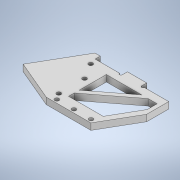
# Autodesk Inventor part: Trunk_lower_side_frame
Saved by Autodesk Inventor 2020.4 (Build 244396000, 396)
## iProperties
Created: 2022-01-02
Part Number: Trunk_lower_side_frame
Material: 一般
Document SubType Name: Modeling
Designer: Masato Kubotera
Density: 1 g/cm^3
Appearance: 既定
Mass: 14.6824 g
Surface Area: 92.1199 cm^2
Volume: 14.6824 cm^3
Author: Masato Kubotera
Autodesk Inventor part; units mm, degrees
ref_plane "YZ Plane" through (0, 0, 0) normal (1, 0, 0) x (0, 1, 0)
ref_plane "XZ Plane" through (0, 0, 0) normal (0, 1, 0) x (-1, 0, 0)
ref_plane "XY Plane" through (0, 0, 0) normal (0, 0, 1) x (1, 0, 0)
derived "Trunk_basis.ipt"
sketch "スケッチ1" plane through (0, 0, 0) normal (0, 1, 0) x (-1, 0, 0)
  line L0 (0, 22) -> (0, -143) construction
  circle A0 centre (5, 0) radius 10.5 construction
  line L1 (-7, 16) -> (36, 16) construction
  line L2 (36, 16) -> (36, -16) construction
  line L3 (36, -16) -> (-7, -16) construction
  line L4 (-7, -16) -> (-7, 16) construction
  line L5 (-7, 16) -> (36, -16) construction
  line L6 (36, 16) -> (-7, -16) construction
  line L7 (33, 13.5) -> (6, 13.5) construction
  line L8 (6, 13.5) -> (6, -13.5) construction
  line L9 (6, -13.5) -> (33, -13.5) construction
  line L10 (33, -13.5) -> (33, 13.5) construction
  line L11 (33, 13.5) -> (6, -13.5) construction
  line L12 (6, 13.5) -> (33, -13.5) construction
  line L13 (-7, 0) -> (36, 0) construction
  arc A1 (5, 16) -> (-7, 10.583) centre (5, 0) ccw construction
  line L14 (34.5651, -16.05) -> (5, -16.05)
  line L15 (5, 16.05) -> (34.5651, 16.05)
  line L16 (36.05, 14.5651) -> (36.05, -14.5651)
  line L17 (36.05, -16.05) -> (-7.05, 16.05) construction
  line L18 (-7.05, -16.05) -> (36.05, 16.05) construction
  arc A2 (5, 16.05) -> (-6.5314, 11.1638) centre (5, 0) ccw
  arc A3 (-6.5314, 11.1638) -> (-7.05, 9.8372) centre (-6.0721, 10.2196) ccw
  arc A4 (36.05, 14.5651) -> (34.5651, 16.05) centre (35.3075, 15.3075) ccw
  circle A5 centre (6, 13.5) radius 1.35 construction
  line L19 (19.5, 13.5) -> (19.5, -13.5) construction
  circle A6 centre (33, 13.5) radius 1.35 construction
  line L20 (-12, 22) -> (-14.5, 19.5)
  line L21 (-14.5, 19.5) -> (-14.5, -13.5)
  line L22 (-14.5, -13.5) -> (-28.5, -27.5)
  line L23 (-28.5, -27.5) -> (-28.5, -97)
  line L24 (52, -13.5) -> (52, 19.5)
  line L25 (52, 19.5) -> (49.5, 22)
  line L26 (49.5, 22) -> (-12, 22)
  line L27 (-28.5, -121.925) -> (-28.5, -139)
  line L28 (-16, -139) -> (-16, -99.5) construction
  line L29 (-16, -99.5) -> (16, -99.5) construction
  line L30 (16, -139) -> (16, -99.5) construction
  line L31 (-7.5, -139) -> (-7.5, -143)
  line L32 (-7.5, -143) -> (7.5, -143)
  line L33 (7.5, -139) -> (7.5, -143)
  arc A7 (-7.5, -139) -> (-9.6, -139) centre (-8.55, -139) ccw
  arc A8 (9.6, -139) -> (7.5, -139) centre (8.55, -139) ccw
  line L34 (-22, -139) -> (-22, -133) construction
  line L35 (-23.5, -133) -> (-20.5, -133) construction
  line L36 (-23.5, -133) -> (-23.5, -139) construction
  line L37 (-20.5, -133) -> (-20.5, -139) construction
  line L38 (-12, 22) -> (-7, 22) construction
  line L39 (-7, 22) -> (-7, -22) construction
  line L40 (-7, -22) -> (-12, -22) construction
  line L41 (-12, -22) -> (-12, 22) construction
  line L42 (-12, 22) -> (-7, -22) construction
  line L43 (-7, 22) -> (-12, -22) construction
  line L44 (-9.5, 22) -> (-9.5, -22) construction
  line L45 (-7, 0) -> (-12, 0) construction
  circle A9 centre (-9.5, 17.75) radius 1.6
  line L46 (-12, 10) -> (-9.5, 10) construction
  line L47 (-9.5, 10) -> (-9.5, -10) construction
  line L48 (-9.5, -10) -> (-12, -10) construction
  line L49 (-12, -10) -> (-12, 10) construction
  line L50 (-12, 10) -> (-9.5, -10) construction
  line L51 (-9.5, 10) -> (-12, -10) construction
  line L52 (-9.45, 10.05) -> (-12.05, 10.05)
  line L53 (-12.05, 7.95) -> (-12.05, -7.95)
  line L54 (-12.05, -10.05) -> (-9.45, -10.05)
  line L55 (-9.45, -7.95) -> (-9.45, 7.95)
  line L56 (-9.45, 10.05) -> (-12.05, -10.05) construction
  line L57 (-12.05, 10.05) -> (-9.45, -10.05) construction
  arc A10 (-12.05, 10.05) -> (-12.05, 7.95) centre (-12.05, 9) ccw
  line L58 (-10.75, 10) -> (-10.75, -10) construction
  arc A11 (-9.45, 7.95) -> (-9.45, 10.05) centre (-9.45, 9) ccw
  circle A12 centre (-9.5, -17.75) radius 1.6
  arc A13 (-12.05, -7.95) -> (-12.05, -10.05) centre (-12.05, -9) ccw
  arc A14 (-9.45, -10.05) -> (-9.45, -7.95) centre (-9.45, -9) ccw
  line L59 (36, 14.4) -> (44.5, 14.4) construction
  line L60 (44.5, 14.4) -> (44.5, -14.4) construction
  line L61 (36, -14.4) -> (44.5, -14.4) construction
  line L62 (46.95, 7.95) -> (46.95, -7.95)
  line L63 (49.5, 0) -> (44.5, 0) construction
  line L64 (44.5, 22) -> (49.5, 22) construction
  line L65 (49.55, -7.95) -> (49.55, 7.95)
  line L66 (48.25, 10) -> (48.25, -10) construction
  line L67 (49.5, 10) -> (47, -10) construction
  line L68 (49.5, -10) -> (47, -10) construction
  line L69 (49.5, 10) -> (49.5, -10) construction
  line L70 (47, 10) -> (49.5, -10) construction
  line L71 (46.95, -10.05) -> (49.55, -10.05)
  line L72 (46.95, 10.05) -> (49.55, -10.05) construction
  line L73 (49.55, 10.05) -> (46.95, -10.05) construction
  line L74 (49.5, -22) -> (44.5, -22) construction
  line L75 (44.5, 22) -> (49.5, -22) construction
  line L76 (49.5, 22) -> (49.5, -22) construction
  line L77 (49.5, 22) -> (44.5, -22) construction
  line L78 (47, 22) -> (47, -22) construction
  line L79 (44.5, -22) -> (44.5, 22) construction
  circle A15 centre (47, -17.75) radius 1.6
  arc A16 (49.55, -10.05) -> (49.55, -7.95) centre (49.55, -9) ccw
  line L80 (47, -10) -> (47, 10) construction
  arc A17 (46.95, -7.95) -> (46.95, -10.05) centre (46.95, -9) ccw
  arc A18 (46.95, 10.05) -> (46.95, 7.95) centre (46.95, 9) ccw
  arc A19 (49.55, 7.95) -> (49.55, 10.05) centre (49.55, 9) ccw
  line L81 (47, 10) -> (49.5, 10) construction
  line L82 (49.55, 10.05) -> (46.95, 10.05)
  circle A20 centre (47, 17.75) radius 1.6
  circle A21 centre (5, 0) radius 16 construction
  arc A22 (-6.5314, -11.1638) -> (5, -16.05) centre (5, 0) ccw
  arc A23 (-7.05, -9.8372) -> (-6.5314, -11.1638) centre (-6.0721, -10.2196) ccw
  arc A24 (34.5651, -16.05) -> (36.05, -14.5651) centre (35.3075, -15.3075) ccw
  line L83 (-7.05, -9.8372) -> (-7.05, 9.8372)
  line L84 (22, -139) -> (22, -133) construction
  line L85 (23.5, -133) -> (23.5, -139) construction
  line L86 (20.5, -133) -> (20.5, -139) construction
  line L87 (23.5, -133) -> (20.5, -133) construction
  circle A25 centre (6, -13.5) radius 1.35
  circle A26 centre (33, -13.5) radius 1.35
  line L88 (188, -110.7642) -> (183, -110.7642)
  line L89 (183, -110.7642) -> (183, -167.2358) construction
  line L90 (183, -167.2358) -> (188, -167.2358) construction
  line L91 (188, -167.2358) -> (188, -110.7642)
  line L92 (188, -110.7642) -> (183, -167.2358) construction
  line L93 (183, -110.7642) -> (188, -167.2358) construction
  line L94 (22, -108.5) -> (56, -108.5) construction
  line L95 (56, -108.5) -> (56, -131.5) construction
  line L96 (56, -131.5) -> (22, -131.5) construction
  line L97 (22, -131.5) -> (22, -108.5) construction
  line L98 (22, -108.5) -> (56, -131.5) construction
  line L99 (56, -108.5) -> (22, -131.5) construction
  line L100 (22, -131.5) -> (52, -131.5) construction
  line L101 (52, -131.5) -> (52, -136.5) construction
  line L102 (52, -136.5) -> (22, -136.5) construction
  line L103 (22, -136.5) -> (22, -131.5) construction
  line L104 (22, -131.5) -> (52, -136.5) construction
  line L105 (52, -131.5) -> (22, -136.5) construction
  line L106 (-25.5, -133) -> (-25.5, -125.2997)
  line L107 (-13.0156, -103.6762) -> (13.8385, -103.6762)
  line L108 (-13.5728, -133) -> (13.8385, -133)
  line L109 (13.8385, -133) -> (13.8385, -111.9605)
  line L110 (13.8385, -111.9605) -> (-13.5728, -133)
  line L111 (22, -99.5) -> (17, -99.5) construction
  line L112 (17, -99.5) -> (17, -123.9917) construction
  line L113 (17, -123.9917) -> (22, -123.9917) construction
  line L114 (22, -123.9917) -> (22, -99.5) construction
  line L115 (22, -99.5) -> (17, -123.9917) construction
  line L116 (17, -99.5) -> (22, -123.9917) construction
  line L117 (19.5, -99.5) -> (19.5, -123.9917) construction
  circle A27 centre (19.5, -101.7459) radius 1.6
  line L118 (17, -111.7459) -> (22, -111.7459) construction
  line L119 (-28.5, -139) -> (-28.5, -143) construction
  line L120 (-28.5, -143) -> (-7.5, -143) construction
  line L121 (28.5, -143) -> (7.5, -143) construction
  line L122 (28.5, -139) -> (28.5, -143) construction
  circle A28 centre (19.5, -121.7459) radius 1.6
  line L123 (17, -106.7459) -> (22, -106.7459) construction
  line L124 (17, -116.7459) -> (22, -116.7459) construction
  line L125 (39.4409, -150.6176) -> (61.7571, -150.6176)
  line L126 (63.242, -152.1025) -> (63.242, -179.9354)
  line L127 (61.7571, -181.4204) -> (39.4409, -181.4204)
  line L128 (37.9559, -179.9354) -> (37.9559, -152.1025)
  line L129 (37.9559, -150.6176) -> (63.242, -181.4204) construction
  line L130 (63.242, -150.6176) -> (37.9559, -181.4204) construction
  arc A29 (39.4409, -150.6176) -> (37.9559, -152.1025) centre (38.6984, -151.36) ccw
  line L131 (50.599, -150.6176) -> (50.599, -181.4204) construction
  line L132 (37.9559, -166.019) -> (63.242, -166.019) construction
  arc A30 (63.242, -152.1025) -> (61.7571, -150.6176) centre (62.4995, -151.36) ccw
  arc A31 (37.9559, -179.9354) -> (39.4409, -181.4204) centre (38.6984, -180.6779) ccw
  arc A32 (61.7571, -181.4204) -> (63.242, -179.9354) centre (62.4995, -180.6779) ccw
  arc A33 (18.4349, -106.6959) -> (16.95, -108.1808) centre (17.6925, -107.4383) ccw
  line L133 (18.4349, -106.6959) -> (20.5651, -106.6959)
  arc A34 (22.05, -108.1808) -> (20.5651, -106.6959) centre (21.3075, -107.4383) ccw
  line L134 (16.95, -115.3109) -> (16.95, -108.1808)
  line L135 (16.95, -111.7459) -> (22.05, -111.7459) construction
  arc A35 (16.95, -115.3109) -> (18.4349, -116.7959) centre (17.6925, -116.0534) ccw
  line L136 (19.5, -106.6959) -> (19.5, -116.7959) construction
  line L137 (16.95, -106.6959) -> (22.05, -116.7959) construction
  line L138 (22.05, -106.6959) -> (16.95, -116.7959) construction
  line L139 (20.5651, -116.7959) -> (18.4349, -116.7959)
  line L140 (22.05, -108.1808) -> (22.05, -115.3109)
  arc A36 (20.5651, -116.7959) -> (22.05, -115.3109) centre (21.3075, -116.0534) ccw
  line L141 (37, -131.5) -> (37, -136.5) construction
  line L142 (32, -131.5) -> (32, -136.5) construction
  line L143 (52, -134) -> (22, -134)
  circle A37 centre (27, -134) radius 1.6
  arc A38 (42.05, -132.9349) -> (40.5651, -131.45) centre (41.3075, -132.1925) ccw
  arc A39 (33.4349, -131.45) -> (31.95, -132.9349) centre (32.6925, -132.1925) ccw
  line L144 (31.95, -134) -> (42.05, -134) construction
  line L145 (33.4349, -131.45) -> (40.5651, -131.45)
  line L146 (42.05, -132.9349) -> (42.05, -135.0651)
  line L147 (40.5651, -136.55) -> (33.4349, -136.55)
  line L148 (31.95, -135.0651) -> (31.95, -132.9349)
  line L149 (31.95, -131.45) -> (42.05, -136.55) construction
  line L150 (42.05, -131.45) -> (31.95, -136.55) construction
  line L151 (37, -131.45) -> (37, -136.55) construction
  arc A40 (31.95, -135.0651) -> (33.4349, -136.55) centre (32.6925, -135.8075) ccw
  arc A41 (40.5651, -136.55) -> (42.05, -135.0651) centre (41.3075, -135.8075) ccw
  line L152 (42, -131.5) -> (42, -136.5) construction
  circle A42 centre (47, -134) radius 1.6
  line L153 (-13.0156, -103.6762) -> (-25.5, -125.2997)
  line L154 (-25.5, -133) -> (-18.5, -133)
  line L155 (-18.5, -133) -> (13.8385, -108.1787)
  line L156 (13.8385, -108.1787) -> (13.8385, -103.6762)
  line L157 (-23.5, -22.5) -> (61, -22.5) construction
  line L158 (52, -13.5) -> (61, -22.5)
  line L159 (61, -22.5) -> (61, -89.5)
  circle A43 centre (-13.5, -58.5) radius 1.75
  line L160 (-18.5, -62.5) -> (51, -62.5)
  line L161 (51, -62.5) -> (51, -90.9057)
  line L162 (51, -90.9057) -> (-18.5, -90.9057)
  line L163 (-18.5, -90.9057) -> (-18.5, -62.5)
  line L164 (-18.5, -62.5) -> (51, -90.9057) construction
  line L165 (51, -62.5) -> (-18.5, -90.9057) construction
  line L166 (-18.5, -27.5) -> (51, -27.5)
  line L167 (51, -27.5) -> (51, -54.5)
  line L168 (51, -54.5) -> (-18.5, -54.5)
  line L169 (-18.5, -54.5) -> (-18.5, -27.5)
  line L170 (-18.5, -27.5) -> (51, -54.5) construction
  line L171 (51, -27.5) -> (-18.5, -54.5) construction
  line L172 (-23.5, -102) -> (-28.5, -97)
  line L173 (-23.5, -99.5) -> (56, -99.5) construction
  line L174 (56, -99.5) -> (56, -94.5) construction
  line L175 (56, -94.5) -> (-23.5, -94.5) construction
  line L176 (-23.5, -94.5) -> (-23.5, -99.5) construction
  line L177 (-23.5, -99.5) -> (56, -94.5) construction
  line L178 (56, -99.5) -> (-23.5, -94.5) construction
  line L179 (-23.5, -97) -> (56, -97) construction
  line L180 (16.25, -94.5) -> (16.25, -99.5) construction
  circle A44 centre (-10.2473, -97) radius 1.6
  circle A45 centre (3.0013, -97) radius 1.6
  circle A46 centre (16.25, -97) radius 1.6
  circle A47 centre (29.4987, -97) radius 1.6
  circle A48 centre (42.7473, -97) radius 1.6
  line L181 (-23.5, -102) -> (15.5276, -102)
  line L182 (15.5276, -102) -> (15.5276, -139)
  line L183 (15.5276, -139) -> (61, -139)
  line L184 (61, -139) -> (61, -94.5)
  line L185 (-28.5, -139) -> (-9.6, -139)
  line L186 (9.6, -139) -> (28.5, -139)
  line L187 (-12.6661, -94.5) -> (22, -94.5)
  line L188 (22, -94.5) -> (53.0898, -107.6708)
  line L189 (53.0898, -107.6708) -> (32.6925, -143)
  line L190 (32.6925, -143) -> (28.55, -143)
  line L191 (28.55, -139) -> (28.55, -143)
  line L192 (-12.6661, -94.5) -> (-28.5, -121.925)
  line L193 (61, -89.5) -> (61, -94.5)
  point P0 (0, 0)
  point P1 (14.5, 0)
  point P2 (19.5, 0)
  point P3 (-7.05, 10.6019)
  point P4 (19.5, 0)
  point P5 (-9.5, 0)
  point P6 (-10.75, 0)
  point P7 (36.05, 14.4)
  point P8 (36.05, -14.4)
  point P9 (48.25, 0)
  point P10 (47, 0)
  point P11 (185.5, -139)
  point P12 (39, -120)
  point P13 (37, -134)
  point P14 (19.5, -111.7459)
  point P15 (50.599, -166.019)
  point P16 (19.5, -111.7459)
  point P17 (19.5, -111.7459)
  point P18 (37, -134)
  point P19 (37, -134)
  point P20 (12.1884, -103.6336)
  point P21 (16.25, -76.7028)
  point P22 (16.25, -41)
  point P23 (30.6126, -98.1486)
  point P24 (27.8987, -96.9989)
  dimension "d4" = 44
  measures "d4" distance of L84.start L34.start
extrude "押し出し1" add sketch "スケッチ1" along normal blind 5 contours L192 L187 L188 A47 L189 L145 A39 L148 A40 L147 L183 L182 L181 | L181 L182 L186 A8 L33 L32 L31 A7 L185 L27 L192 | L189 L190 L191 L183 | L188 A47 | L147 A40 L148 L143 L189 | L143 L148 A39 L145 L189 | L133 A34 L140 A36 L139 A35 L134 A33 picked at (29.2737, -97.9903)
